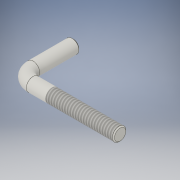
# Autodesk Inventor part: fc17-015_AnchorBolt
Saved by Autodesk Inventor 2017.1 (Build 211199000, 199)
## iProperties
Category: Screws
Company: Autodesk Inc.
Created: 2016-12-15
Part Number: fc17-015_AnchorBolt
Material: Steel
Document SubType Name: Modeling
Designer: Autodesk Inc.
Density: 7.85 g/cm^3
Appearance: Steel
Catalog Web Link: http://firstchoicebyandymark.com/fc17-015
Vendor: AndyMark Inc.
Author: Autodesk Inc.
Keywords: FIRST Choice
Autodesk Inventor part; units mm, degrees
ref_plane "YZ Plane" through (0, 0, 0) normal (1, 0, 0) x (0, 1, 0)
ref_plane "XZ Plane" through (0, 0, 0) normal (0, 1, 0) x (-1, 0, 0)
ref_plane "XY Plane" through (0, 0, 0) normal (0, 0, 1) x (1, 0, 0)
sketch "Sketch1" plane through (0, 0, 0) normal (0, 1, 0) x (-1, 0, 0)
  line L0 (0, 0) -> (41.275, 0)
  line L1 (47.625, -6.35) -> (47.625, -25.4)
  arc A0 (47.625, -6.35) -> (41.275, 0) centre (41.275, -6.35) ccw
  point P0 (47.625, 0)
  dimension "d0" = 47.625
  dimension "d1" = 25.4
  dimension "d3" = 6.35
  constraints: 4 end point, 2 point on circle, 2 point on line, 2 tangent, 1 centre point, 1 horizontal, 1 perpendicular
  measures "d0" distance of L0.start point (47.625, 0)
  measures "d1" distance of point (47.625, 0) L1.end
  measures "d3" radius of A0
sketch "Sketch2" plane through (0, 0, 0) normal (1, 0, 0) x (0, 1, 0)
  circle A0 centre (0, 0) radius 3.175
  dimension "d2" = 6.35
  constraints: 1 centre point, 1 coincident
  measures "d2" diameter of A0
sweep "Sweep1" add profiles "Sketch2" path "Sketch1"
chamfer "Chamfer1" distance 0.508 angle 45 1 edges at (0, -3.175, 0)
thread "Thread1"
chamfer "Chamfer2" distance 0.508 angle 45 1 edges at (-47.625, -3.175, -25.4)
body "Solid1"
